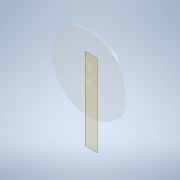
# Autodesk Inventor part: szklo
Saved by Autodesk Inventor 2021 (Build 250183000, 183)
## iProperties
Created: 2021-11-16
Part Number: szklo
Material: Akrylowy, przezroczysty
Document SubType Name: Modeling
Designer: wojwo
Density: 1.19 g/cm^3
Appearance: Przezroczyste — przejrzyste
Author: wojwo
Autodesk Inventor part; units mm, degrees
ref_plane "YZ Plane" through (0, 0, 0) normal (1, 0, 0) x (0, 1, 0)
ref_plane "XZ Plane" through (0, 0, 0) normal (0, 1, 0) x (-1, 0, 0)
ref_plane "XY Plane" through (0, 0, 0) normal (0, 0, 1) x (1, 0, 0)
ref_plane "Płaszczyzna konstrukcyjna1" through (0, 0, 0) normal (0, 0, 1) x (1, 0, 0)
sketch "Szkic1" plane through (0, 0, 0) normal (0, 0, 1) x (1, 0, 0)
  circle A0 centre (0, 20) radius 2.5 projected
  circle A1 centre (0, 35) radius 2.5 projected
  circle A2 centre (0, 27.5) radius 40
  point P0 (0, 0)
  dimension "d0" = 7.5
  dimension "d1" = 7.5
  dimension "d2" = 80
  constraints: 1 centre point, 1 coincident
  measures "d0" distance of A0.centre point (0, 27.5)
  measures "d1" distance of A1.centre point (0, 27.5)
  measures "d2" diameter of A2
extrude "Wyciągnięcie proste1" add sketch "Szkic1" along normal blind 3
chamfer "Faza1" distance 0.4 angle 45 2 edges at (-40, 27.5, 3) (-40, 27.5, 0)
chamfer "Faza3" distance 2 angle 45 2 edges at (-2.5, 20, 3) (-2.5, 35, 3)
sketch "Szkic2" plane through (0, 27.5, 0) normal (0, 0, -1) x (-1, 0, 0)
  circle A0 centre (0, 7.5) radius 2.5 projected
  circle A1 centre (0, -7.5) radius 2.5 projected
  circle A2 centre (0, -47.5) radius 2 projected
  circle A3 centre (0, -62.5) radius 2 projected
  line L0 (6.05, 12.2) -> (6.05, -67.2) projected
  line L1 (-6.05, 12.2) -> (6.05, 12.2) projected
  line L2 (-6.05, -67.2) -> (-6.05, 12.2) projected
  line L3 (6.05, -67.2) -> (-6.05, -67.2) projected
  circle A4 centre (0, 7.5) radius 2.5 projected
  circle A5 centre (0, -7.5) radius 2.5 projected
  circle A6 centre (0, -47.5) radius 2 projected
  circle A7 centre (0, -62.5) radius 2 projected
  line L4 (6.05, 12.2) -> (6.05, -67.2) projected
  line L5 (-6.05, 12.2) -> (6.05, 12.2) projected
  line L6 (-6.05, -67.2) -> (-6.05, 12.2) projected
  line L7 (6.05, -67.2) -> (-6.05, -67.2) projected
  line L8 (10, -41.5) -> (-10, -41.5)
  line L9 (-10, -41.5) -> (-10, -15.5)
  line L10 (-8, -13.5) -> (8, -13.5)
  line L11 (10, -15.5) -> (10, -41.5)
  line L12 (10, -41.5) -> (-10, -13.5) construction
  line L13 (-10, -41.5) -> (10, -13.5) construction
  arc A8 (-8, -13.5) -> (-10, -15.5) centre (-8, -15.5) ccw
  arc A9 (10, -15.5) -> (8, -13.5) centre (8, -15.5) ccw
  point P0 (0, -27.5)
  point P1 (0, -27.5)
  dimension "d14" = 20
  dimension "d15" = 28
  dimension "d16" = 20
  dimension "d17" = 2
  constraints: 12 end point, 4 point on circle, 4 point on line, 4 tangent, 2 centre point, 2 midpoint, 2 parallel, 1 equal radius, 1 horizontal, 1 perpendicular
  measures "d14" distance of L12.end L13.end
  measures "d15" distance of L8.end L12.end
  measures "d16" distance of point (0, -27.5) A1.centre
  measures "d17" radius of A8
extrude "Wyciągnięcie proste2" cut sketch "Szkic2" against normal blind 2 contours L10 A9 L11 L8 L0 | L0 L8 L2 L10 | L2 L8 L9 A8 L10
